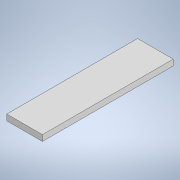
# Autodesk Inventor part: FP Chassis
Saved by Autodesk Inventor 2020 (Build 240168000, 168)
## iProperties
Created: 2021-04-14
Part Number: FP Chassis
Material: Generic
Document SubType Name: Modeling
Designer: austi
Density: 1 g/cm^3
Appearance: Default
Author: austi
Autodesk Inventor part; units mm, degrees
ref_plane "YZ Plane" through (0, 0, 0) normal (1, 0, 0) x (0, 1, 0)
ref_plane "XZ Plane" through (0, 0, 0) normal (0, 1, 0) x (-1, 0, 0)
ref_plane "XY Plane" through (0, 0, 0) normal (0, 0, 1) x (1, 0, 0)
sketch "Sketch1" plane through (0, 0, 0) normal (0, 1, 0) x (-1, 0, 0)
  line L0 (21, 0) -> (-21, 0) projected
  line L1 (0, -77) -> (0, 77) projected
  line L2 (15, 55) -> (-15, 55)
  line L3 (-15, 55) -> (-15, -55)
  line L4 (-15, -55) -> (15, -55)
  line L5 (15, -55) -> (15, 55)
  point P0 (0, 0)
  point P1 (15, 0)
  point P2 (0, 55)
  dimension "d0" = 30
  dimension "d1" = 110
  constraints: 8 end point, 2 midpoint, 2 parallel, 1 horizontal, 1 horizontal alignment, 1 perpendicular, 1 vertical alignment
  measures "d0" distance of L4.end L3.end
  measures "d1" distance of L3.end L2.end
extrude "Extrusion1" add sketch "Sketch1" along normal blind 5
body "Solid1"
